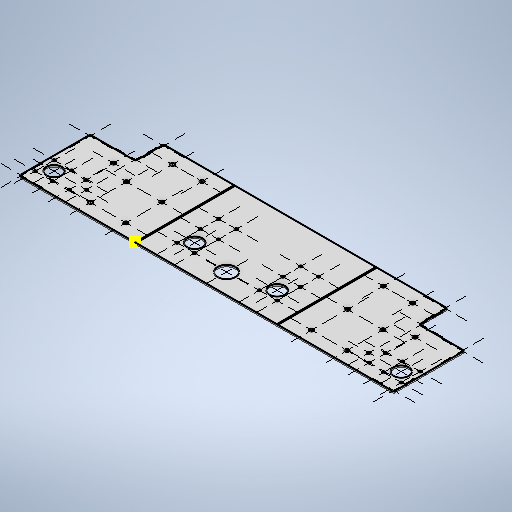
# Autodesk Inventor part: body_main_frame
Saved by Autodesk Inventor 2026.1 (Build 301233000, 233)
## iProperties
Created: 2025-08-15
Part Number: body_main_frame
Material: Generic
Document SubType Name: Modeling
Designer: chris
Density: 1 g/cm^3
Appearance: Default
Author: chris
Autodesk Inventor part; units mm, degrees
ref_plane "YZ Plane" through (0, 0, 0) normal (1, 0, 0) x (0, 1, 0)
ref_plane "XZ Plane" through (0, 0, 0) normal (0, 1, 0) x (-1, 0, 0)
ref_plane "XY Plane" through (0, 0, 0) normal (0, 0, 1) x (1, 0, 0)
sketch "Sketch1" plane through (0, 0, 0) normal (0, 1, 0) x (-1, 0, 0)
  line L0 (-0.4496, -84) -> (-0.4496, 0)
  line L1 (-120.7289, 0) -> (-120.7289, -84)
  circle A0 centre (-60.5893, -17) radius 7.5
  circle A1 centre (-25.6593, -25) radius 6.5
  circle A2 centre (-95.5193, -25) radius 6.5
  circle A3 centre (-18.1343, -17.5) radius 1.05
  circle A4 centre (-18.1343, -37.5) radius 1.05
  circle A5 centre (-18.1343, -52.6) radius 1.05
  circle A6 centre (-33.1843, -52.6) radius 1.05
  circle A7 centre (-33.1843, -37.5) radius 1.05
  circle A8 centre (-33.1843, -17.5) radius 1.05
  circle A9 centre (-87.9943, -17.5) radius 1.05
  circle A10 centre (-87.9943, -37.5) radius 1.05
  circle A11 centre (-87.9943, -52.6) radius 1.05
  circle A12 centre (-103.0443, -52.6) radius 1.05
  circle A13 centre (-103.0443, -37.5) radius 1.05
  circle A14 centre (-103.0443, -17.5) radius 1.05
  circle A15 centre (-215.8686, -26) radius 1.05
  circle A16 centre (94.69, -26) radius 1.05
  circle A17 centre (-215.8686, -9.86) radius 1.05
  circle A18 centre (94.69, -9.86) radius 1.05
  circle A19 centre (-207.8686, -17.93) radius 6.4
  circle A20 centre (86.69, -17.93) radius 6.4
  circle A21 centre (-188.4636, -49.095) radius 1.55
  circle A22 centre (67.285, -49.095) radius 1.55
  circle A23 centre (-137.4636, -73.095) radius 1.55
  circle A24 centre (16.285, -73.095) radius 1.55
  circle A25 centre (-162.4636, -73.095) radius 1.55
  circle A26 centre (41.285, -73.095) radius 1.55
  circle A27 centre (-139.3686, -40.905) radius 1.55
  circle A28 centre (18.19, -40.905) radius 1.55
  circle A29 centre (-169.3686, -40.905) radius 1.55
  circle A30 centre (48.19, -40.905) radius 1.55
  circle A31 centre (-139.3686, -10.405) radius 1.55
  circle A32 centre (18.19, -10.405) radius 1.55
  circle A33 centre (-169.3686, -10.405) radius 1.55
  circle A34 centre (48.19, -10.405) radius 1.55
  circle A35 centre (-200.9686, -9.93) radius 1.05
  circle A36 centre (-200.9686, -25.93) radius 1.05
  circle A37 centre (-187.7486, -24.93) radius 1.05
  circle A38 centre (-180.4486, -17.93) radius 1.05
  circle A39 centre (-187.7486, -10.93) radius 1.05
  circle A40 centre (79.79, -9.93) radius 1.05
  circle A41 centre (79.79, -25.93) radius 1.05
  circle A42 centre (66.57, -24.93) radius 1.05
  circle A43 centre (59.27, -17.93) radius 1.05
  circle A44 centre (66.57, -10.93) radius 1.05
  arc A45 (-219.3686, -59) -> (-218.3686, -60) centre (-218.3686, -59) ccw
  line L2 (-218.3686, -60) -> (-181.8686, -60)
  arc A46 (-180.8686, -61) -> (-181.8686, -60) centre (-181.8686, -61) ccw
  arc A47 (-180.8686, -83) -> (-179.8686, -84) centre (-179.8686, -83) ccw
  line L3 (-180.8686, -61) -> (-180.8686, -83)
  arc A48 (58.69, -84) -> (59.69, -83) centre (58.69, -83) ccw
  line L4 (59.69, -83) -> (59.69, -61)
  arc A49 (60.69, -60) -> (59.69, -61) centre (60.69, -61) ccw
  line L5 (60.69, -60) -> (97.19, -60)
  arc A50 (97.19, -60) -> (98.19, -59) centre (97.19, -59) ccw
  line L6 (98.19, -1) -> (98.19, -59)
  arc A51 (98.19, -1) -> (97.19, 0) centre (97.19, -1) ccw
  line L7 (-218.3686, 0) -> (97.19, 0)
  arc A52 (-218.3686, 0) -> (-219.3686, -1) centre (-218.3686, -1) ccw
  line L8 (-219.3686, -59) -> (-219.3686, -1)
  line L9 (58.69, -84) -> (-179.8686, -84)
  line L10 (-121.1786, -84) -> (-121.1786, 0)
  line L11 (-120.2793, 0) -> (-120.2793, -84)
  line L12 (-0.8993, -84) -> (-0.8993, 0)
  line L13 (0, 0) -> (0, -84)
  point P0 (0, 0)
  constraints: 53 centre point, 47 equal radius, 28 end point, 17 tangent, 16 point on circle, 12 point on line, 10 vertical, 9 parallel, 4 horizontal, 3 perpendicular, 135 other
extrude "Extrusion1" add sketch "Sketch1" against normal blind 1.5
body "Solid1"
